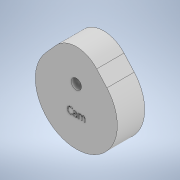
# Autodesk Inventor part: Cam
Saved by Autodesk Inventor 2021 (Build 250183000, 183)
## iProperties
Created: 2021-04-12
Part Number: Cam
Material: Generic
Document SubType Name: Modeling
Designer: Nabeel Azafer
Density: 1 g/cm^3
Appearance: Default
Mass: 3.73641 g
Surface Area: 16.6071 cm^2
Volume: 3.73641 cm^3
Author: Nabeel Azafer
Autodesk Inventor part; units mm, degrees
note: some values were not read from the file. Chosen so that the rebuilt part matches the saved one: direction of "Emboss1".
ref_plane "YZ Plane" through (0, 0, 0) normal (1, 0, 0) x (0, 1, 0)
ref_plane "XZ Plane" through (0, 0, 0) normal (0, 1, 0) x (-1, 0, 0)
ref_plane "XY Plane" through (0, 0, 0) normal (0, 0, 1) x (1, 0, 0)
sketch "Sketch1" plane through (0, 0, 0) normal (0, 0, 1) x (1, 0, 0)
  arc A0 (-8.9443, 8) -> (8.9443, 8) centre (0, 0) ccw
  arc A1 (5.9628, 11.3333) -> (-5.9628, 11.3333) centre (0, 6) ccw
  line L0 (-5.9628, 11.3333) -> (-8.9443, 8)
  line L1 (5.9628, 11.3333) -> (8.9443, 8)
  circle A2 centre (0, 4.5) radius 2.5
  point P0 (1, 2.2087)
  dimension "d3" = 5
  dimension "d0" = 24
  dimension "d1" = 6
  dimension "d2" = 16
  dimension "d4" = 4.5
  constraints: 4 end point, 4 point on circle, 4 tangent, 2 centre point, 1 coincident, 3 other
  measures "d0" diameter of A0
  measures "d1" distance of point (0, 0) A1.centre
  measures "d2" diameter of A1
  measures "d4" distance of point (0, 0) point (0, 4.5)
extrude "Extrusion1" add sketch "Sketch1" along normal blind 8 contours L0 A1 L1 A0 | A2
sketch "Sketch2" plane through (0, 0, 8) normal (0, 0, 1) x (1, 0, 0)
  line L0 (-2.6829, -1.9742) -> (11.2377, -1.9742) construction
  line L1 (11.2377, -1.9742) -> (11.2377, -6.0238) construction
  line L2 (11.2377, -6.0238) -> (-2.6829, -6.0238) construction
  line L3 (-2.6829, -6.0238) -> (-2.6829, -1.9742) construction
  spline S0 degree 2 poles (-1.6991, -4.0455) (-1.8936, -4.0455) (-2.2226, -3.9142) (-2.3425, -3.7829) knots 0 0 0 1 2 2 2
  spline S1 degree 2 poles (-2.3425, -3.7829) (-2.4625, -3.6533) (-2.5937, -3.2643) (-2.5937, -3.0115) knots 0 0 0 1 2 2 2
  spline S2 degree 2 poles (-2.5937, -3.0115) (-2.5937, -2.7603) (-2.4657, -2.3875) (-2.3441, -2.2497) knots 0 0 0 1 2 2 2
  spline S3 degree 2 poles (-2.3441, -2.2497) (-2.2242, -2.1152) (-1.8968, -1.9742) (-1.6942, -1.9742) knots 0 0 0 1 2 2 2
  spline S4 degree 2 poles (-1.6942, -1.9742) (-1.5937, -1.9742) (-1.4171, -2.0034) (-1.3425, -2.0261) knots 0 0 0 1 2 2 2
  spline S5 degree 2 poles (-1.3425, -2.0261) (-1.2777, -2.0471) (-1.1432, -2.1071) (-1.0767, -2.1428) knots 0 0 0 1 2 2 2
  line L4 (-1.0767, -2.1428) -> (-1.0767, -2.4637)
  line L5 (-1.0767, -2.4637) -> (-1.0978, -2.4637)
  spline S6 degree 2 poles (-1.0978, -2.4637) (-1.1335, -2.4312) (-1.2437, -2.3405) (-1.3231, -2.2967) knots 0 0 0 1 2 2 2
  spline S7 degree 2 poles (-1.3231, -2.2967) (-1.3993, -2.2546) (-1.5792, -2.2011) (-1.6958, -2.2011) knots 0 0 0 1 2 2 2
  spline S8 degree 2 poles (-1.6958, -2.2011) (-1.8239, -2.2011) (-2.0524, -2.3065) (-2.1383, -2.4069) knots 0 0 0 1 2 2 2
  spline S9 degree 2 poles (-2.1383, -2.4069) (-2.2226, -2.509) (-2.3166, -2.8186) (-2.3166, -3.0115) knots 0 0 0 1 2 2 2
  spline S10 degree 2 poles (-2.3166, -3.0115) (-2.3166, -3.2173) (-2.2177, -3.5139) (-2.1318, -3.616) knots 0 0 0 1 2 2 2
  spline S11 degree 2 poles (-2.1318, -3.616) (-2.0476, -3.7149) (-1.8223, -3.8154) (-1.6958, -3.8154) knots 0 0 0 1 2 2 2
  spline S12 degree 2 poles (-1.6958, -3.8154) (-1.5808, -3.8154) (-1.3847, -3.7586) (-1.3085, -3.7165) knots 0 0 0 1 2 2 2
  spline S13 degree 2 poles (-1.3085, -3.7165) (-1.2356, -3.6744) (-1.127, -3.5868) (-1.0962, -3.556) knots 0 0 0 1 2 2 2
  line L6 (-1.0962, -3.556) -> (-1.0767, -3.556)
  line L7 (-1.0767, -3.556) -> (-1.0767, -3.8737)
  spline S14 degree 2 poles (-1.0767, -3.8737) (-1.1432, -3.9045) (-1.2599, -3.9612) (-1.3425, -3.9872) knots 0 0 0 1 2 2 2
  spline S15 degree 2 poles (-1.3425, -3.9872) (-1.43, -4.0163) (-1.5792, -4.0455) (-1.6991, -4.0455) knots 0 0 0 1 2 2 2
  spline S16 degree 2 poles (-0.0119, -3.851) (-0.0427, -3.8737) (-0.1464, -3.9547) (-0.195, -3.9791) knots 0 0 0 1 2 2 2
  spline S17 degree 2 poles (-0.195, -3.9791) (-0.2615, -4.0147) (-0.3863, -4.052) (-0.4997, -4.052) knots 0 0 0 1 2 2 2
  spline S18 degree 2 poles (-0.4997, -4.052) (-0.5921, -4.052) (-0.7591, -3.9823) (-0.8223, -3.9191) knots 0 0 0 1 2 2 2
  spline S19 degree 2 poles (-0.8223, -3.9191) (-0.8822, -3.8575) (-0.9552, -3.676) (-0.9552, -3.5755) knots 0 0 0 1 2 2 2
  spline S20 degree 2 poles (-0.9552, -3.5755) (-0.9552, -3.4199) (-0.8239, -3.1995) (-0.6813, -3.1363) knots 0 0 0 1 2 2 2
  spline S21 degree 2 poles (-0.6813, -3.1363) (-0.5548, -3.0779) (-0.2112, -3.0342) (-0.0119, -3.0228) knots 0 0 0 1 2 2 2
  line L8 (-0.0119, -3.0228) -> (-0.0119, -2.9742)
  spline S22 degree 2 poles (-0.0119, -2.9742) (-0.0119, -2.8867) (-0.0654, -2.7781) (-0.114, -2.7473) knots 0 0 0 1 2 2 2
  spline S23 degree 2 poles (-0.114, -2.7473) (-0.1626, -2.7165) (-0.302, -2.697) (-0.3766, -2.697) knots 0 0 0 1 2 2 2
  spline S24 degree 2 poles (-0.3766, -2.697) (-0.4641, -2.697) (-0.7007, -2.7489) (-0.819, -2.7992) knots 0 0 0 1 2 2 2
  line L9 (-0.819, -2.7992) -> (-0.8336, -2.7992)
  line L10 (-0.8336, -2.7992) -> (-0.8336, -2.5415)
  spline S25 degree 2 poles (-0.8336, -2.5415) (-0.7639, -2.522) (-0.503, -2.4734) (-0.3749, -2.4734) knots 0 0 0 1 2 2 2
  spline S26 degree 2 poles (-0.3749, -2.4734) (-0.2194, -2.4734) (-0.007, -2.522) (0.0772, -2.5852) knots 0 0 0 1 2 2 2
  spline S27 degree 2 poles (0.0772, -2.5852) (0.1599, -2.6468) (0.2409, -2.8429) (0.2409, -2.9839) knots 0 0 0 1 2 2 2
  line L11 (0.2409, -2.9839) -> (0.2409, -4.0099)
  line L12 (0.2409, -4.0099) -> (-0.0119, -4.0099)
  line L13 (-0.0119, -4.0099) -> (-0.0119, -3.851)
  line L14 (-0.0119, -3.6403) -> (-0.0119, -3.2238)
  spline S28 degree 2 poles (-0.0119, -3.2238) (-0.1027, -3.2319) (-0.3766, -3.2594) (-0.4625, -3.2854) knots 0 0 0 1 2 2 2
  spline S29 degree 2 poles (-0.4625, -3.2854) (-0.5629, -3.3162) (-0.6942, -3.4442) (-0.6942, -3.5577) knots 0 0 0 1 2 2 2
  spline S30 degree 2 poles (-0.6942, -3.5577) (-0.6942, -3.6873) (-0.5484, -3.8186) (-0.409, -3.8186) knots 0 0 0 1 2 2 2
  spline S31 degree 2 poles (-0.409, -3.8186) (-0.2907, -3.8186) (-0.0962, -3.7165) (-0.0119, -3.6403) knots 0 0 0 1 2 2 2
  line L15 (2.2977, -4.0099) -> (2.2977, -3.1411)
  spline S32 degree 2 poles (2.2977, -3.1411) (2.2977, -3.0374) (2.2815, -2.8607) (2.2555, -2.8121) knots 0 0 0 1 2 2 2
  spline S33 degree 2 poles (2.2555, -2.8121) (2.2296, -2.7586) (2.1307, -2.7068) (2.0448, -2.7068) knots 0 0 0 1 2 2 2
  spline S34 degree 2 poles (2.0448, -2.7068) (1.967, -2.7068) (1.7888, -2.8024) (1.6948, -2.8932) knots 0 0 0 1 2 2 2
  spline S35 degree 2 poles (1.6948, -2.8932) (1.6964, -2.9159) (1.6996, -2.9791) (1.6996, -3.0212) knots 0 0 0 1 2 2 2
  line L16 (1.6996, -3.0212) -> (1.6996, -4.0099)
  line L17 (1.6996, -4.0099) -> (1.4468, -4.0099)
  line L18 (1.4468, -4.0099) -> (1.4468, -3.1411)
  spline S36 degree 2 poles (1.4468, -3.1411) (1.4468, -3.0374) (1.4306, -2.8607) (1.4046, -2.8121) knots 0 0 0 1 2 2 2
  spline S37 degree 2 poles (1.4046, -2.8121) (1.3787, -2.7586) (1.2798, -2.7068) (1.1939, -2.7068) knots 0 0 0 1 2 2 2
  spline S38 degree 2 poles (1.1939, -2.7068) (1.1129, -2.7068) (0.933, -2.8089) (0.8487, -2.8883) knots 0 0 0 1 2 2 2
  line L19 (0.8487, -2.8883) -> (0.8487, -4.0099)
  line L20 (0.8487, -4.0099) -> (0.5959, -4.0099)
  line L21 (0.5959, -4.0099) -> (0.5959, -2.509)
  line L22 (0.5959, -2.509) -> (0.8487, -2.509)
  line L23 (0.8487, -2.509) -> (0.8487, -2.6744)
  spline S39 degree 2 poles (0.8487, -2.6744) (0.9476, -2.5755) (1.1421, -2.4669) (1.2588, -2.4669) knots 0 0 0 1 2 2 2
  spline S40 degree 2 poles (1.2588, -2.4669) (1.3917, -2.4669) (1.5975, -2.5885) (1.651, -2.7262) knots 0 0 0 1 2 2 2
  spline S41 degree 2 poles (1.651, -2.7262) (1.7661, -2.5982) (1.9832, -2.4669) (2.1097, -2.4669) knots 0 0 0 1 2 2 2
  spline S42 degree 2 poles (2.1097, -2.4669) (2.2069, -2.4669) (2.3657, -2.5269) (2.4241, -2.5949) knots 0 0 0 1 2 2 2
  spline S43 degree 2 poles (2.4241, -2.5949) (2.4841, -2.663) (2.5505, -2.8672) (2.5505, -3.0212) knots 0 0 0 1 2 2 2
  line L24 (2.5505, -3.0212) -> (2.5505, -4.0099)
  line L25 (2.5505, -4.0099) -> (2.2977, -4.0099)
  point P0 (0, 0)
  constraints: 2 other
emboss "Emboss1" sketch "Sketch2" operation cut depth 1 direction (0, 0, -1)
sketch "Sketch3" plane through (0, 0, 8) normal (0, 0, 1) x (1, 0, 0)
  circle A0 centre (0, 4.5) radius 2.5
  point P0 (0, 0)
  dimension "d11" = 5
  dimension "d12" = 4.5
  constraints: 1 centre point
  measures "d11" diameter of A0
  measures "d12" distance of point (0, 0) A0.centre
hole "Hole1" at (0, 4.5, 8) direction (0, 0, -1) diameter 3 end through all
body "Solid1"
